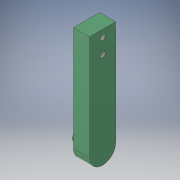
# Autodesk Inventor part: Arm2
Saved by Autodesk Inventor 2018 (Build 220112000, 112)
## iProperties
Created: 2018-09-18
Part Number: Arm2
Material: Generic
Document SubType Name: Modeling
Designer: Viraj Shah
Density: 1 g/cm^3
Appearance: Default
Mass: 5.91105 g
Surface Area: 27.6709 cm^2
Volume: 5.91105 cm^3
Author: Viraj Shah
Autodesk Inventor part; units mm, degrees
ref_plane "YZ Plane" through (0, 0, 0) normal (1, 0, 0) x (0, 1, 0)
ref_plane "XZ Plane" through (0, 0, 0) normal (0, 1, 0) x (-1, 0, 0)
ref_plane "XY Plane" through (0, 0, 0) normal (0, 0, 1) x (1, 0, 0)
sketch "Sketch1" plane through (0, 0, 0) normal (1, 0, 0) x (0, 1, 0)
  line L0 (6.5194, -26.4952) -> (6.5, 25.5048)
  line L1 (6.5, 25.5048) -> (-6.5, 25.5)
  line L2 (-6.5, 25.5) -> (-6.4806, -26.5)
  line L3 (-6.4806, -26.5) -> (6.5, 25.5048) construction
  line L4 (6.5194, -26.4952) -> (-6.5, 25.5) construction
  circle A0 centre (-0.0034, 14.5024) radius 1.25
  arc A1 (-6.4806, -26.5) -> (6.5194, -26.4952) centre (0.0194, -26.4976) ccw
  circle A2 centre (-0.0017, 22.0024) radius 1.25
  dimension "d8" = 13
  dimension "d12" = 2.5
  dimension "d22" = 52
  dimension "d23" = 6.5
  dimension "d24" = 90
  dimension "d25" = 90
  dimension "d26" = 11
  dimension "d27" = 2.5
  dimension "d28" = 7.5
  constraints: 10 end point, 3 centre point, 2 point on circle, 1 parallel
  measures "d8" distance of L1.end L0.end
  measures "d12" diameter of A0
  measures "d22" distance of L1.end L2.end
  measures "d23" radius of A1
  measures "d24" angle of L1 L0
  measures "d25" angle of L2 L1
  measures "d26" distance from line of L1 A0.centre
  measures "d27" diameter of A2
  measures "d28" distance of A0.centre A2.centre
extrude "Extrusion1" add sketch "Sketch1" along normal blind 8
sketch "Sketch2" plane through (0, 0, 0) normal (-1, 0, 0) x (0, 0, 1)
  arc A0 (-26.4952, 6.5194) -> (-26.5, -6.4806) centre (-26.4976, 0.0194) ccw projected
  circle A1 centre (-26.4976, 0.0194) radius 1.5
  point P0 (0, 0)
  dimension "d16" = 3
  constraints: 1 centre point
  measures "d16" diameter of A1
extrude "Extrusion2" add sketch "Sketch2" along normal blind 3
sketch "Sketch3" plane through (-3, 0.0194, -26.4976) normal (-1, 0, 0) x (0, 0, 1)
  circle A0 centre (0, 0) radius 1.5 projected
  circle A1 centre (0, 0) radius 2.5
  point P0 (26.4976, -0.0194)
  dimension "d19" = 5
  constraints: 1 centre point, 1 coincident
  measures "d19" diameter of A1
extrude "Extrusion3" add sketch "Sketch3" along normal blind 1.5 contours A0 | A1
body "Solid1"
